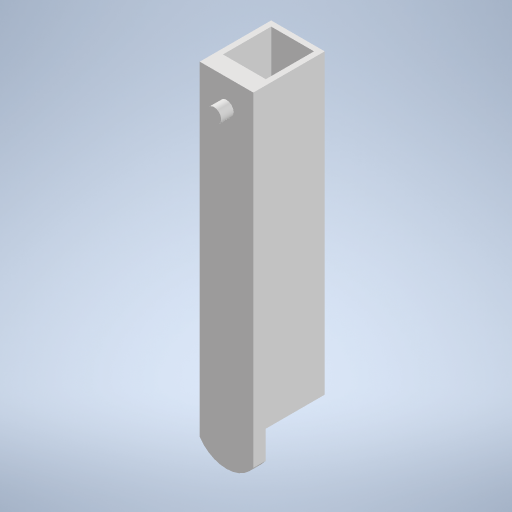
# Autodesk Inventor part: arm1
Saved by Autodesk Inventor 2024 (Build 280153000, 153)
## iProperties
Created: 2025-11-24
Part Number: arm1
Material: Generic
Document SubType Name: Modeling
Designer: Aidan
Density: 1 g/cm^3
Appearance: Default
Author: Aidan
Autodesk Inventor part; units mm, degrees
ref_plane "YZ Plane" through (0, 0, 0) normal (1, 0, 0) x (0, 1, 0)
ref_plane "XZ Plane" through (0, 0, 0) normal (0, 1, 0) x (-1, 0, 0)
ref_plane "XY Plane" through (0, 0, 0) normal (0, 0, 1) x (1, 0, 0)
sketch "Sketch1" plane through (0, 0, 0) normal (0, 0, 1) x (1, 0, 0)
  line L0 (0, 0) -> (30, 0)
  line L1 (30, 0) -> (30, 200)
  line L2 (30, 200) -> (0, 200)
  line L3 (0, 200) -> (0, 0)
  dimension "d0" = 30
  dimension "d1" = 200
  constraints: 8 end point, 2 parallel, 1 horizontal, 1 perpendicular
  measures "d0" distance of L2.end L1.end
  measures "d1" distance of L1.end L0.end
extrude "Extrusion1" add sketch "Sketch1" along normal blind 40
sketch "Sketch2" plane through (0, 0, 0) normal (-1, 0, 0) x (0, 0, 1)
  line L0 (0, 0) -> (33, 0)
  line L1 (33, 0) -> (33, 33.5)
  line L2 (33, 33.5) -> (0, 33.5)
  line L3 (0, 33.5) -> (0, 0)
  dimension "d4" = 33
  dimension "d5" = 33.5
  constraints: 8 end point, 2 parallel, 1 horizontal, 1 perpendicular
  measures "d4" distance of L2.end L1.end
  measures "d5" distance of L1.end L0.end
extrude "Extrusion2" cut sketch "Sketch2" against normal up to surface (30 mm away)
sketch "Sketch3" plane through (0, 0, 33) normal (0, 0, -1) x (-1, 0, 0)
  circle A0 centre (-15, 18) radius 3.95
  line L0 (0, 0) -> (-30, 0) projected
  line L1 (0, 33.5) -> (0, 0) projected
  dimension "d8" = 7.9
  dimension "d9" = 18
  dimension "d10" = 15
  constraints: 1 centre point
  measures "d8" diameter of A0
  measures "d9" distance from line of L0 A0.centre
  measures "d10" distance from line of L1 A0.centre
extrude "Extrusion3" add sketch "Sketch3" along normal blind 7
sketch "Sketch5" plane through (0, 0, 40) normal (0, 0, 1) x (1, 0, 0)
  line L0 (0, 33.5) -> (0, 0) projected
  line L1 (30, 0) -> (30, 200) projected
  line L2 (0, 0) -> (30, 0)
  line L3 (30, 0) -> (30, 10)
  line L4 (30, 10) -> (0, 10)
  line L5 (0, 10) -> (0, 0)
  dimension "d16" = 10
  constraints: 8 end point, 2 parallel, 1 horizontal, 1 perpendicular, 1 point on line
  measures "d16" distance of L3.end L2.end
extrude "Extrusion5" cut sketch "Sketch5" against normal up to surface (7 mm away)
sketch "Sketch7" plane through (0, 0, 40) normal (0, 0, 1) x (1, 0, 0)
  circle A0 centre (15, 185) radius 4
  line L0 (30, 200) -> (0, 200) projected
  line L1 (30, 10) -> (30, 200) projected
  point P0 (0, 0)
  dimension "d19" = 8
  dimension "d22" = 15
  dimension "d23" = 15
  constraints: 1 centre point
  measures "d19" diameter of A0
  measures "d22" distance from line of L0 A0.centre
  measures "d23" distance from line of L1 A0.centre
extrude "Extrusion6" add sketch "Sketch7" along normal blind 7
sketch "Sketch8" plane through (0, 33.5, 0) normal (0, -1, 0) x (1, 0, 0)
  line L0 (30, 33) -> (30, 0) projected
  line L1 (0, 33) -> (30, 33) projected
  line L2 (0, 0) -> (0, 33) projected
  line L3 (30, 0) -> (0, 0) projected
  line L4 (3, 30) -> (27, 30)
  line L5 (27, 30) -> (27, 3)
  line L6 (27, 3) -> (3, 3)
  line L7 (3, 3) -> (3, 30)
  point P0 (0, 0)
  dimension "d24" = 3
  constraints: 8 end point, 3 other
  measures "d24" distance between parallel lines of L2 L7
extrude "Extrusion7" cut sketch "Sketch8" against normal up to surface (166.5 mm away) contours L4 L5 L6 L7
sketch "Sketch9" plane through (0, 0, 40) normal (0, 0, 1) x (1, 0, 0)
  circle A0 centre (15, 18) radius 3.95 projected
  line L0 (0, 200) -> (0, 10) projected
  line L1 (30, 10) -> (30, 33.5) projected
  arc A1 (0, 18) -> (30, 18) centre (15, 28.0625) ccw
  line L2 (30, 10) -> (0, 10) projected
  line L3 (0, 18) -> (0, 10)
  line L4 (0, 10) -> (30, 10)
  line L5 (30, 18) -> (30, 10)
  line L6 (15, 18) -> (15, 28.0625) construction
  point P0 (0, 0)
  point P1 (15, 10)
  dimension "d27" = 8
  constraints: 8 end point, 3 collinear, 2 point on circle, 2 point on line, 1 centre point, 1 tangent, 1 vertical
  measures "d27" distance from line of L3.start L2
extrude "Extrusion8" cut sketch "Sketch9" against normal up to surface (7 mm away) contours A1 L2 L0 | A1 L1 L2
body "Solid1"
